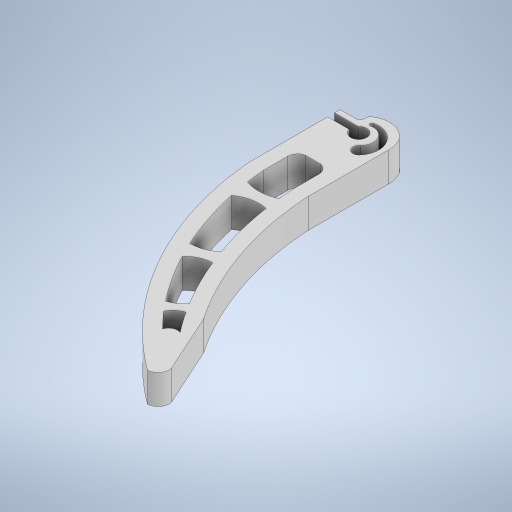
# Autodesk Inventor part: Central Claw_Exterior claw  V3
Saved by Autodesk Inventor 2024 (Build 280153000, 153)
## iProperties
Created: 2025-03-24
Part Number: Central Claw_Exterior claw  V3
Material: Generic
Document SubType Name: Modeling
Designer: b_arm
Density: 1 g/cm^3
Appearance: Default
Author: b_arm
## iProperties of the stored document Central Claw V2_3DPrint.ipt
Created: 2025-03-24
Part Number: Central Claw V2_3DPrint
Material: Generic
Document SubType Name: Modeling
Designer: b_arm
Density: 1 g/cm^3
Appearance: Default
Author: b_arm
Autodesk Inventor part; units mm, degrees
ref_plane "YZ Plane" through (0, 0, 0) normal (1, 0, 0) x (0, 1, 0)
ref_plane "XZ Plane" through (0, 0, 0) normal (0, 1, 0) x (-1, 0, 0)
ref_plane "XY Plane" through (0, 0, 0) normal (0, 0, 1) x (1, 0, 0)
sketch "Sketch1" plane through (0, 0, 0) normal (0, 1, 0) x (-1, 0, 0)
  arc A0 (3.9007, 1.0556) -> (2.1982, -3.3894) centre (0.0024, 0.0001) ccw
  arc A1 (19.0232, 1.0556) -> (-16.4856, -9.5418) centre (0.0024, 0.0001) ccw
  line L0 (3.9007, 1.0556) -> (19.0232, 1.0556)
  line L1 (2.1982, -3.3894) -> (19.0232, -3.3894)
  line L2 (19.0232, -7.0431) -> (11.658, -7.0431)
  line L3 (19.0232, -3.3894) -> (19.0232, -7.0431)
  arc A2 (-16.4856, -9.5418) -> (7.4534, -10.991) centre (-3.9181, -0.3889) ccw
  line L4 (19.0232, 1.0556) -> (19.0232, 51.8556)
  line L5 (-19.0476, 0.0001) -> (-19.0476, 51.8556)
  line L6 (-19.0476, 0.0001) -> (-19.4605, 0.0001)
  arc A3 (19.0232, 51.8556) -> (-64.3153, 200.5038) centre (-187.3249, 33.8538) ccw
  arc A4 (-19.0476, 51.5998) -> (-53.7472, 153.729) centre (-221.3606, 39.8209) ccw
  line L7 (9.8792, 51.4484) -> (9.8792, 35.8565)
  arc A5 (-10.1576, 51.8556) -> (-53.8573, 169.027) centre (-221.3606, 39.8209) ccw
  line L8 (-10.1576, 51.8556) -> (-10.1576, 35.8565)
  line L9 (9.8792, 23.8284) -> (-10.1576, 23.8284) construction
  line L10 (9.8792, 23.8284) -> (29.9159, 23.8284) construction
  arc A6 (4.8483, 29.6451) -> (9.8792, 35.8565) centre (3.5292, 35.8565) ccw
  arc A7 (-10.1576, 35.8565) -> (-5.1267, 29.6451) centre (-3.8076, 35.8565) ccw
  line L11 (4.8483, 29.6451) -> (-5.1267, 29.6451)
  arc A8 (19.0232, 51.8556) -> (-64.3153, 200.5038) centre (-187.3249, 33.8538) ccw
  arc A9 (-31.6355, 156.1642) -> (-40.7288, 149.9287) centre (-26.0329, 138.2456) ccw
  arc A10 (-25.3873, 119.4827) -> (-11.9806, 125.796) centre (-26.0329, 138.2456) ccw
  arc A11 (-7.259, 116.1658) -> (-22.0111, 110.6115) centre (-7.259, 93.7981) ccw
  arc A12 (-12.2768, 72.0005) -> (6.1478, 75.8935) centre (-7.259, 93.7981) ccw
  arc A13 (8.4637, 63.2789) -> (-11.0177, 62.3465) centre (-0.1392, 39.0411) ccw
  arc A14 (-44.388, 155.7184) -> (-36.6502, 162.2912) centre (-47.9514, 167.7544) ccw
  line L12 (7.4534, -9.5831) -> (7.4534, -10.991)
  line L13 (11.658, -7.0431) -> (9.9934, -7.0431)
  line L14 (9.9934, -7.0431) -> (7.4534, -7.0431)
  line L15 (7.4534, -7.0431) -> (7.4534, -9.5831)
  line L16 (-53.7472, 153.729) -> (-70.9133, 191.6752)
  arc A15 (-64.3153, 200.5038) -> (-70.9133, 191.6752) centre (-63.9188, 193.3277) ccw
  arc A16 (-53.8573, 169.027) -> (-46.1861, 172.7021) centre (-51.6725, 174.3104) ccw
  arc A17 (9.8792, 51.4484) -> (-46.1861, 172.7021) centre (-187.3249, 33.8538) ccw
  point P0 (-0.1392, 29.6451)
  point P1 (19.0232, 1.0556)
  point P2 (-64.3153, 200.5038)
  point P3 (7.4534, 1.0556)
  dimension "d17" = 8.0772
  dimension "d19" = 4.445
  dimension "d22" = 50.8
  dimension "d27" = 8.89
  dimension "d28" = 8.89
  dimension "d31" = 180
  dimension "d32" = 6.35
  dimension "d33" = 207.1318
  dimension "d34" = 33.8537
  dimension "d35" = 29.6449
  dimension "d36" = 19.05
  dimension "d37" = 3.3895
  constraints: 51 point on circle, 34 end point, 18 centre point, 6 horizontal, 5 point on line, 4 perpendicular, 3 vertical, 2 equal radius, 2 tangent, 1 coincident, 1 collinear, 1 midpoint
  measures "d17" diameter of A0
  measures "d19" distance between parallel lines of L1 L0
  measures "d22" distance of L4.start L4.end
  measures "d27" radial gap between concentric circles of A4 A5
  measures "d28" distance between parallel lines of L5 L8
  measures "d31" angle of L9 L10
  measures "d32" radius of A6
  measures "d33" radius of A3
  measures "d34" vertical distance of A0.centre A3.centre
  measures "d35" vertical distance of A0.centre point (-0.139, 29.645)
  measures "d36" radius of A1
  measures "d37" distance from line of A1.centre L1
extrude "Extrusion1" add sketch "Sketch1" along normal blind 19.05 contours A0 L1 L3 L2 L13 L14 L15 L12 A2 A1 L0 | A1 L5 A4 L16 A15 A3 L4 | A13 A5 A12 A17 | A11 A5 A10 A17 | A9 A5 A14 A17
fillet "Fillet1" radius 1.27 1 edges at (-7.4534, 9.525, -7.0431)
sketch "Sketch2" plane through (-19.0232, 0, -7.0431) normal (0, 0, -1) x (-1, 0, 0)
  line L0 (0, 0) -> (0, 19.05) projected
  line L1 (-10.2998, 19.05) -> (0, 19.05) projected
  point P0 (-19.0232, 0)
  point P1 (-5.08, 9.525)
  point P2 (0, 9.525)
  point P3 (-5.1499, 19.05)
  dimension "d44" = 5.08
  dimension "d45" = 9.525
  constraints: 2 midpoint
  measures "d44" distance of point (0, 9.525) point (-5.08, 9.525)
  measures "d45" vertical distance of point (-5.15, 19.05) point (-5.08, 9.525)
hole "Hole1" at (-13.9432, 9.525, -7.0431) direction (0, 0, 1) diameter 5.334 end up to surface
sketch "Sketch3" plane through (-3.9007, 0, 1.0556) normal (0, 0, -1) x (-1, 0, 0)
  circle A0 centre (10.0425, 9.525) radius 2.667 projected
  point P0 (-3.9007, 0)
  constraints: 1 coincident
hole "Hole2" at (-13.9432, 9.525, 1.0556) direction (0, 0, 1) diameter 5.588 depth 10.16
sketch "Sketch4" plane through (-19.0232, 0, 1.0556) normal (-1, 0, 0) x (0, 0, 1)
  line L0 (0, 6.731) -> (0, 12.319) projected
  line L1 (10.16, 12.319) -> (10.16, 6.731) projected
  line L2 (0, 6.731) -> (5.08, 6.731)
  line L3 (10.16, 6.731) -> (0, 6.731) projected
  line L4 (0, 12.319) -> (5.08, 12.319)
  line L5 (10.16, 12.319) -> (0, 12.319) projected
  line L6 (0, 0) -> (50.8, 0) projected
  line L7 (0, 9.525) -> (16.1442, 9.525) construction
  line L8 (5.08, 9.525) -> (5.08, 2.921)
  line L9 (5.08, 9.525) -> (5.08, 16.129)
  line L10 (5.08, 16.129) -> (22.86, 16.129)
  line L11 (22.86, 16.129) -> (22.86, 2.921)
  line L12 (22.86, 2.921) -> (5.08, 2.921)
  point P0 (-1.0556, 0)
  dimension "d63" = 5.08
  dimension "d65" = 6.604
  dimension "d66" = 6.604
  dimension "d67" = 17.78
  constraints: 16 end point, 3 midpoint, 3 perpendicular, 2 vertical, 1 horizontal, 1 point on line
  measures "d63" distance of L0.start L2.end
  measures "d65" distance of L8.start L8.end
  measures "d66" distance of L8.start L9.end
  measures "d67" distance of L9.end L10.end
extrude "Extrusion2" cut sketch "Sketch4" against normal blind 11.43 contours L8 L9 L5 L1 L3 | L3 L1 L5 L9 L10 L11 L12 L8
sketch "Sketch6" plane through (0, 0, 0) normal (0, -1, 0) x (1, 0, 0)
  circle A0 centre (-0.4283, -8.8611) radius 1.27
  circle A1 centre (9.6886, 9.5689) radius 3.81
  arc A2 (-0.3421, -7.594) -> (6.8398, 7.039) centre (0.2554, 1.1917) ccw
  arc A3 (-0.7205, -10.097) -> (12.5379, 12.0984) centre (2.3988, 3.0973) ccw
  arc A4 (-7.4534, -10.991) -> (16.4856, -9.5418) centre (3.9181, -0.3889) ccw projected
  line L0 (-9.198, -6.9778) -> (-6.15, -6.9778)
  line L1 (-6.15, -6.9778) -> (-6.15, -12.2358)
  line L2 (-6.15, -12.2358) -> (-9.198, -12.2358)
  line L3 (-9.198, -12.2358) -> (-9.198, -6.9778)
  point P0 (0, 0)
  dimension "d90" = 3.048
  dimension "d91" = 2.54
  constraints: 9 point on circle, 8 end point, 4 centre point, 4 tangent, 2 parallel, 1 horizontal, 1 perpendicular, 1 other
  measures "d90" distance of L1.end L2.end
  measures "d91" diameter of A0
extrude "Extrusion4" cut sketch "Sketch6" against normal blind 25.4
fillet "Fillet2" radius 3.175 1 edges at (-6.15, 9.525, -6.9778)
fillet "Fillet3" radius 3.175 1 edges at (-6.15, 9.525, -12.2358)
sketch "Sketch7" plane through (0, 0, 0) normal (0, -1, 0) x (1, 0, 0)
  circle A0 centre (0, 0) radius 5.1181
  dimension "d96" = 10.2362
  constraints: 1 centre point, 1 coincident
  measures "d96" diameter of A0
extrude "FOR EXTERIOR" cut sketch "Sketch7" against normal blind 25.4
sketch "Sketch8" plane through (0, 0, 0) normal (0, -1, 0) x (1, 0, 0)
  arc A0 (-3.835, -3.3894) -> (-5.0081, 1.0556) centre (0, 0) ccw projected
  arc A1 (-0.3421, -7.594) -> (6.8398, 7.039) centre (0.2554, 1.1917) ccw projected
  arc A2 (12.5379, 12.0984) -> (6.8398, 7.039) centre (9.6886, 9.5689) ccw projected
  arc A3 (-0.7205, -10.097) -> (12.5379, 12.0984) centre (2.3988, 3.0973) ccw projected
  arc A4 (-0.3421, -7.594) -> (-0.7205, -10.097) centre (-0.4283, -8.8611) ccw projected
  circle A5 centre (9.6886, 9.5689) radius 3.81
  circle A6 centre (-0.4283, -8.8611) radius 1.27
  arc A7 (-0.3421, -7.594) -> (6.8398, 7.039) centre (1.573, 0.545) ccw
  point P0 (0.0088, -7.6687)
  point P1 (7.474, 6.4687)
  point P2 (6.8398, 7.039)
  point P3 (-0.3421, -7.594)
  constraints: 3 centre point, 2 coincident, 2 point on circle, 1 concentric
extrude "For Exterior claw" add sketch "Sketch8" against normal up to surface (19.05 mm away) contours A1 A5 A7 A6
sketch "Sketch9" plane through (0, 0, 0) normal (0, -1, 0) x (1, 0, 0)
  point P0 (0, 0)
body "Solid1"
